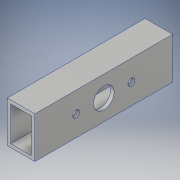
# Autodesk Inventor part: 2AM-17-P-5209 - cylinder mount
Saved by Autodesk Inventor 2017 (Build 210142000, 142)
## iProperties
Created: 2017-09-30
Part Number: 2AM-17-P-5209 - cylinder mount
Material: Aluminum 6061
Document SubType Name: Modeling
Designer: Gus
Density: 2.7 g/cm^3
Appearance: Aluminum - Flat
Mass: 90.2705 g
Surface Area: 223.851 cm^2
Volume: 33.4335 cm^3
Author: Gus
Autodesk Inventor part; units mm, degrees
ref_plane "YZ Plane" through (0, 0, 0) normal (1, 0, 0) x (0, 1, 0)
ref_plane "XZ Plane" through (0, 0, 0) normal (0, 1, 0) x (-1, 0, 0)
ref_plane "XY Plane" through (0, 0, 0) normal (0, 0, 1) x (1, 0, 0)
sketch "Sketch1" plane through (0, 0, 0) normal (0, 0, 1) x (1, 0, 0)
  line L0 (-12.7, -19.05) -> (12.7, -19.05)
  line L1 (12.7, -19.05) -> (12.7, 19.05)
  line L2 (12.7, 19.05) -> (-12.7, 19.05)
  line L3 (-12.7, 19.05) -> (-12.7, -19.05)
  line L4 (-12.7, -19.05) -> (12.7, 19.05) construction
  line L5 (12.7, -19.05) -> (-12.7, 19.05) construction
  line L6 (-9.525, 15.875) -> (9.525, 15.875)
  line L7 (9.525, 15.875) -> (9.525, -15.875)
  line L8 (9.525, -15.875) -> (-9.525, -15.875)
  line L9 (-9.525, -15.875) -> (-9.525, 15.875)
  point P0 (0, 0)
  dimension "d0" = 25.4
  dimension "d1" = 38.1
  dimension "d2" = 3.175
  constraints: 20 end point, 4 parallel, 2 midpoint, 2 perpendicular, 1 horizontal, 3 other
  measures "d0" distance of L2.end L1.end
  measures "d1" distance of L1.end L0.end
  measures "d2" distance between parallel lines of L2 L6
extrude "Extrusion1" add sketch "Sketch1" along normal mid plane 127
sketch "Sketch2" plane through (12.7, -19.05, 63.5) normal (1, 0, 0) x (0, 0, -1)
  circle A0 centre (63.5, 19.05) radius 3.175
  dimension "d5" = 6.35
  constraints: 1 centre point, 1 coincident
  measures "d5" diameter of A0
extrude "Extrusion2" cut sketch "Sketch2" against normal through all
pattern_linear "Rectangular Pattern1" count 4 spacing 25.4 along (0, 0, 1) of "Extrusion2" first direction both ways yes skipped copies 4
hole "Hole1" at (12.7, 0, 0) direction (-1, 0, 0) diameter 15.875 end through all
hole "Hole2" at (12.7, 0, 0) direction (-1, 0, 0) diameter 19.05 end through all
body "Solid1"
